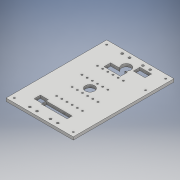
# Autodesk Inventor part: 一枚目
Saved by Autodesk Inventor 2018 (Build 220112000, 112)
## iProperties
Created: 2018-08-15
Part Number: 一枚目
Material: 一般
Document SubType Name: Modeling
Designer: shun2
Density: 1 g/cm^3
Appearance: 既定
Author: shun2
Autodesk Inventor part; units mm, degrees
(part 1 of 2)
ref_plane "YZ Plane" through (0, 0, 0) normal (1, 0, 0) x (0, 1, 0)
ref_plane "XZ Plane" through (0, 0, 0) normal (0, 1, 0) x (-1, 0, 0)
ref_plane "XY Plane" through (0, 0, 0) normal (0, 0, 1) x (1, 0, 0)
sketch "スケッチ2" plane through (0, 0, 0) normal (0, 0, 1) x (1, 0, 0)
  line L0 (0.0414, 0.0414) -> (130.0414, 0.0414)
  line L1 (130.0414, 0.0414) -> (130.0414, 194.7653)
  line L2 (130.0414, 194.7653) -> (0.0414, 194.7653)
  line L3 (0.0414, 194.7653) -> (0.0414, 0.0414)
  circle A0 centre (78.0414, 186.7653) radius 2.15
  circle A1 centre (92.0414, 186.7653) radius 2.15
  circle A2 centre (52.0414, 186.7653) radius 2.15
  circle A3 centre (38.0414, 186.7653) radius 2.15
  circle A4 centre (78.0414, 8.0414) radius 2.15
  circle A5 centre (92.0414, 8.0414) radius 2.15
  circle A6 centre (52.0414, 8.0414) radius 2.15
  circle A7 centre (38.0414, 8.0414) radius 2.15
  circle A8 centre (95.5414, 52.4033) radius 1.6
  circle A9 centre (45.5414, 52.4033) radius 1.6
  circle A10 centre (55.5414, 52.4033) radius 1.6
  circle A11 centre (65.5414, 52.4033) radius 1.6
  circle A12 centre (75.5414, 52.4033) radius 1.6
  circle A13 centre (85.5414, 52.4033) radius 1.6
  circle A14 centre (95.5414, 82.4033) radius 1.6
  circle A15 centre (45.5414, 82.4033) radius 1.6
  circle A16 centre (55.5414, 82.4033) radius 1.6
  circle A17 centre (65.5414, 82.4033) radius 1.6
  circle A18 centre (75.5414, 82.4033) radius 1.6
  circle A19 centre (85.5414, 82.4033) radius 1.6
  circle A20 centre (34.5414, 142.4033) radius 1.6
  circle A21 centre (84.5414, 142.4033) radius 1.6
  circle A22 centre (74.5414, 142.4033) radius 1.6
  circle A23 centre (64.5414, 142.4033) radius 1.6
  circle A24 centre (54.5414, 142.4033) radius 1.6
  circle A25 centre (44.5414, 142.4033) radius 1.6
  circle A26 centre (34.5414, 112.4033) radius 1.6
  circle A27 centre (84.5414, 112.4033) radius 1.6
  circle A28 centre (74.5414, 112.4033) radius 1.6
  circle A29 centre (64.5414, 112.4033) radius 1.6
  circle A30 centre (54.5414, 112.4033) radius 1.6
  circle A31 centre (44.5414, 112.4033) radius 1.6
  circle A32 centre (8.0414, 186.7653) radius 1.6
  circle A33 centre (122.0414, 186.7653) radius 1.6
  circle A34 centre (122.0414, 8.0414) radius 1.6
  circle A35 centre (8.0414, 8.0414) radius 1.6
  circle A36 centre (122.0414, 147.7653) radius 1.6
  line L4 (130.0414, 194.7653) -> (0.0414, 194.7653)
  line L5 (0.0414, 194.7653) -> (0.0414, 0.0414)
  line L6 (0.0414, 0.0414) -> (130.0414, 0.0414)
  line L7 (130.0414, 0.0414) -> (130.0414, 194.7653)
  circle A37 centre (92.0414, 186.7653) radius 2.15
  circle A38 centre (78.0414, 186.7653) radius 2.15
  circle A39 centre (52.0414, 186.7653) radius 2.15
  circle A40 centre (38.0414, 186.7653) radius 2.15
  circle A41 centre (92.0414, 8.0414) radius 2.15
  circle A42 centre (78.0414, 8.0414) radius 2.15
  circle A43 centre (52.0414, 8.0414) radius 2.15
  circle A44 centre (38.0414, 8.0414) radius 2.15
  circle A45 centre (84.5414, 142.4033) radius 1.6
  circle A46 centre (74.5414, 142.4033) radius 1.6
  circle A47 centre (64.5414, 142.4033) radius 1.6
  circle A48 centre (54.5414, 142.4033) radius 1.6
  circle A49 centre (44.5414, 142.4033) radius 1.6
  circle A50 centre (34.5414, 142.4033) radius 1.6
  circle A51 centre (84.5414, 112.4033) radius 1.6
  circle A52 centre (74.5414, 112.4033) radius 1.6
  circle A53 centre (64.5414, 112.4033) radius 1.6
  circle A54 centre (54.5414, 112.4033) radius 1.6
  circle A55 centre (44.5414, 112.4033) radius 1.6
  circle A56 centre (34.5414, 112.4033) radius 1.6
  circle A57 centre (95.5414, 82.4033) radius 1.6
  circle A58 centre (85.5414, 82.4033) radius 1.6
  circle A59 centre (75.5414, 82.4033) radius 1.6
  circle A60 centre (65.5414, 82.4033) radius 1.6
  circle A61 centre (55.5414, 82.4033) radius 1.6
  circle A62 centre (45.5414, 82.4033) radius 1.6
  circle A63 centre (95.5414, 52.4033) radius 1.6
  circle A64 centre (85.5414, 52.4033) radius 1.6
  circle A65 centre (75.5414, 52.4033) radius 1.6
  circle A66 centre (65.5414, 52.4033) radius 1.6
  circle A67 centre (55.5414, 52.4033) radius 1.6
  circle A68 centre (45.5414, 82.4033) radius 1.6
  circle A69 centre (45.5414, 52.4033) radius 1.6
  circle A70 centre (8.0414, 186.7653) radius 1.6
  circle A71 centre (122.0414, 186.7653) radius 1.6
  circle A72 centre (122.0414, 147.7653) radius 1.6
  circle A73 centre (122.0414, 8.0414) radius 1.6
  circle A74 centre (8.0414, 8.0414) radius 1.6
  arc A75 (69.6765, 160.0343) -> (65, 176.7239) centre (65, 167.7239) ccw
  arc A76 (65, 176.7239) -> (60.3235, 160.0343) centre (65, 167.7239) ccw
  line L8 (83.4433, 173.4847) -> (95.4433, 173.4847)
  arc A77 (95.4433, 173.453) -> (95.4433, 173.5164) centre (95.4433, 173.4847) ccw
  arc A78 (83.4433, 173.5164) -> (83.4433, 173.453) centre (83.4433, 173.4847) ccw
  line L9 (95.4433, 173.4847) -> (95.4433, 176.9847)
  arc A79 (95.4751, 176.9847) -> (95.4116, 176.9847) centre (95.4434, 176.9847) ccw
  arc A80 (95.4116, 173.4847) -> (95.4751, 173.4847) centre (95.4434, 173.4847) ccw
  line L10 (95.4433, 176.9847) -> (83.4433, 176.9847)
  arc A81 (83.4433, 177.0164) -> (83.4433, 176.953) centre (83.4433, 176.9847) ccw
  arc A82 (95.4433, 176.953) -> (95.4433, 177.0164) centre (95.4433, 176.9847) ccw
  line L11 (83.4433, 176.9847) -> (83.4433, 173.4847)
  arc A83 (83.4116, 173.4847) -> (83.4751, 173.4847) centre (83.4434, 173.4847) ccw
  arc A84 (83.4751, 176.9847) -> (83.4116, 176.9847) centre (83.4434, 176.9847) ccw
  line L12 (56.515, 150.7744) -> (56.515, 152.1714)
  arc A85 (56.5531, 152.1714) -> (56.4769, 152.1714) centre (56.515, 152.1714) ccw
  arc A86 (56.4769, 150.7744) -> (56.5531, 150.7744) centre (56.515, 150.7744) ccw
  line L13 (46.355, 158.2674) -> (56.515, 158.2674)
  arc A87 (56.515, 158.2293) -> (56.515, 158.3055) centre (56.515, 158.2674) ccw
  arc A88 (46.355, 158.3055) -> (46.355, 158.2293) centre (46.355, 158.2674) ccw
  line L14 (46.355, 158.2674) -> (46.355, 156.4894)
  arc A89 (46.3169, 156.4894) -> (46.3931, 156.4894) centre (46.355, 156.4894) ccw
  arc A90 (46.3931, 158.2674) -> (46.3169, 158.2674) centre (46.355, 158.2674) ccw
  line L15 (56.515, 150.7744) -> (46.355, 150.7744)
  arc A91 (46.355, 150.8125) -> (46.355, 150.7363) centre (46.355, 150.7744) ccw
  arc A92 (56.515, 150.7363) -> (56.515, 150.8125) centre (56.515, 150.7744) ccw
  line L16 (56.515, 157.3784) -> (57.023, 157.5054)
  arc A93 (57.0322, 157.4684) -> (57.0138, 157.5424) centre (57.023, 157.5054) ccw
  arc A94 (56.5058, 157.4154) -> (56.5242, 157.3414) centre (56.515, 157.3784) ccw
  line L17 (56.515, 157.3784) -> (56.515, 158.2674)
  arc A95 (56.5531, 158.2674) -> (56.4769, 158.2674) centre (56.515, 158.2674) ccw
  arc A96 (56.4769, 157.3784) -> (56.5531, 157.3784) centre (56.515, 157.3784) ccw
  line L18 (57.023, 157.5054) -> (57.023, 156.3624)
  arc A97 (56.9849, 156.3624) -> (57.0611, 156.3624) centre (57.023, 156.3624) ccw
  arc A98 (57.0611, 157.5054) -> (56.9849, 157.5054) centre (57.023, 157.5054) ccw
  line L19 (57.023, 156.3624) -> (56.515, 156.4894)
  arc A99 (56.5242, 156.5264) -> (56.5058, 156.4524) centre (56.515, 156.4894) ccw
  arc A100 (57.0138, 156.3254) -> (57.0322, 156.3994) centre (57.023, 156.3624) ccw
  line L20 (56.515, 156.4894) -> (56.515, 157.3784)
  arc A101 (56.5531, 157.3784) -> (56.4769, 157.3784) centre (56.515, 157.3784) ccw
  arc A102 (56.4769, 156.4894) -> (56.5531, 156.4894) centre (56.515, 156.4894) ccw
  line L21 (56.515, 156.4894) -> (46.355, 156.4894)
  arc A103 (46.355, 156.5275) -> (46.355, 156.4513) centre (46.355, 156.4894) ccw
  arc A104 (56.515, 156.4513) -> (56.515, 156.5275) centre (56.515, 156.4894) ccw
  line L22 (46.355, 156.4894) -> (46.355, 152.1714)
  arc A105 (46.3169, 152.1714) -> (46.3931, 152.1714) centre (46.355, 152.1714) ccw
  arc A106 (46.3931, 156.4894) -> (46.3169, 156.4894) centre (46.355, 156.4894) ccw
  line L23 (56.515, 152.1714) -> (46.355, 152.1714)
  arc A107 (46.355, 152.2095) -> (46.355, 152.1333) centre (46.355, 152.1714) ccw
  arc A108 (56.515, 152.1333) -> (56.515, 152.2095) centre (56.515, 152.1714) ccw
  line L24 (56.515, 152.1714) -> (56.515, 156.4894)
  arc A109 (56.5531, 156.4894) -> (56.4769, 156.4894) centre (56.515, 156.4894) ccw
  arc A110 (56.4769, 152.1714) -> (56.5531, 152.1714) centre (56.515, 152.1714) ccw
  line L25 (46.355, 152.1714) -> (46.355, 150.7744)
  arc A111 (46.3169, 150.7744) -> (46.3931, 150.7744) centre (46.355, 150.7744) ccw
  arc A112 (46.3931, 152.1714) -> (46.3169, 152.1714) centre (46.355, 152.1714) ccw
  line L26 (60.565, 151.81) -> (60.565, 156.89)
  arc A113 (60.5968, 156.89) -> (60.5333, 156.89) centre (60.5651, 156.89) ccw
  arc A114 (60.5333, 151.81) -> (60.5968, 151.81) centre (60.5651, 151.81) ccw
  line L27 (60.565, 156.89) -> (61.835, 156.89)
  arc A115 (61.835, 156.8583) -> (61.835, 156.9218) centre (61.835, 156.8901) ccw
  arc A116 (60.565, 156.9218) -> (60.565, 156.8583) centre (60.565, 156.8901) ccw
  line L28 (61.835, 156.89) -> (69.455, 156.89)
  arc A117 (69.455, 156.8583) -> (69.455, 156.9218) centre (69.455, 156.8901) ccw
  arc A118 (61.835, 156.9218) -> (61.835, 156.8583) centre (61.835, 156.8901) ccw
  line L29 (69.455, 156.89) -> (70.725, 156.89)
  arc A119 (70.725, 156.8583) -> (70.725, 156.9218) centre (70.725, 156.8901) ccw
  arc A120 (69.455, 156.9218) -> (69.455, 156.8583) centre (69.455, 156.8901) ccw
  line L30 (70.725, 156.89) -> (70.725, 151.81)
  arc A121 (70.6933, 151.81) -> (70.7568, 151.81) centre (70.725, 151.81) ccw
  arc A122 (70.7568, 156.89) -> (70.6933, 156.89) centre (70.725, 156.89) ccw
  line L31 (70.725, 151.81) -> (60.565, 151.81)
  arc A123 (60.565, 151.8417) -> (60.565, 151.7783) centre (60.565, 151.81) ccw
  arc A124 (70.725, 151.7783) -> (70.725, 151.8417) centre (70.725, 151.81) ccw
  line L32 (61.835, 156.89) -> (61.835, 155.62)
  arc A125 (61.8032, 155.62) -> (61.8668, 155.62) centre (61.835, 155.62) ccw
  arc A126 (61.8668, 156.89) -> (61.8032, 156.89) centre (61.835, 156.89) ccw
  line L33 (61.835, 155.62) -> (69.455, 155.62)
  arc A127 (69.455, 155.5883) -> (69.455, 155.6517) centre (69.455, 155.62) ccw
  arc A128 (61.835, 155.6517) -> (61.835, 155.5883) centre (61.835, 155.62) ccw
  line L34 (69.455, 155.62) -> (69.455, 156.89)
  arc A129 (69.4868, 156.89) -> (69.4232, 156.89) centre (69.455, 156.89) ccw
  arc A130 (69.4232, 155.62) -> (69.4868, 155.62) centre (69.455, 155.62) ccw
  arc A131 (93.9433, 174.5922) -> (93.9433, 175.1172) centre (93.9433, 174.8547) ccw
  arc A132 (93.9433, 175.1172) -> (93.9433, 174.5922) centre (93.9433, 174.8547) ccw
  arc A133 (93.9433, 174.5922) -> (93.9433, 175.1172) centre (93.9433, 174.8547) ccw
  arc A134 (93.9433, 175.1172) -> (93.9433, 174.5922) centre (93.9433, 174.8547) ccw
  arc A135 (92.4433, 174.5922) -> (92.4433, 175.1172) centre (92.4433, 174.8547) ccw
  arc A136 (92.4433, 175.1172) -> (92.4433, 174.5922) centre (92.4433, 174.8547) ccw
  arc A137 (92.4433, 174.5922) -> (92.4433, 175.1172) centre (92.4433, 174.8547) ccw
  arc A138 (92.4433, 175.1172) -> (92.4433, 174.5922) centre (92.4433, 174.8547) ccw
  arc A139 (90.9433, 174.5922) -> (90.9433, 175.1172) centre (90.9433, 174.8547) ccw
  arc A140 (90.9433, 175.1172) -> (90.9433, 174.5922) centre (90.9433, 174.8547) ccw
  arc A141 (90.9433, 174.5922) -> (90.9433, 175.1172) centre (90.9433, 174.8547) ccw
  arc A142 (90.9433, 175.1172) -> (90.9433, 174.5922) centre (90.9433, 174.8547) ccw
  arc A143 (89.4433, 174.5922) -> (89.4433, 175.1172) centre (89.4433, 174.8547) ccw
  arc A144 (89.4433, 175.1172) -> (89.4433, 174.5922) centre (89.4433, 174.8547) ccw
  arc A145 (89.4433, 174.5922) -> (89.4433, 175.1172) centre (89.4433, 174.8547) ccw
  arc A146 (89.4433, 175.1172) -> (89.4433, 174.5922) centre (89.4433, 174.8547) ccw
  arc A147 (87.9433, 174.5922) -> (87.9433, 175.1172) centre (87.9433, 174.8547) ccw
  arc A148 (87.9433, 175.1172) -> (87.9433, 174.5922) centre (87.9433, 174.8547) ccw
  arc A149 (87.9433, 174.5922) -> (87.9433, 175.1172) centre (87.9433, 174.8547) ccw
  arc A150 (87.9433, 175.1172) -> (87.9433, 174.5922) centre (87.9433, 174.8547) ccw
  arc A151 (86.4433, 174.5922) -> (86.4433, 175.1172) centre (86.4433, 174.8547) ccw
  arc A152 (86.4433, 175.1172) -> (86.4433, 174.5922) centre (86.4433, 174.8547) ccw
  arc A153 (86.4433, 174.5922) -> (86.4433, 175.1172) centre (86.4433, 174.8547) ccw
  arc A154 (86.4433, 175.1172) -> (86.4433, 174.5922) centre (86.4433, 174.8547) ccw
  arc A155 (84.9433, 174.5922) -> (84.9433, 175.1172) centre (84.9433, 174.8547) ccw
  arc A156 (84.9433, 175.1172) -> (84.9433, 174.5922) centre (84.9433, 174.8547) ccw
  arc A157 (84.9433, 174.5922) -> (84.9433, 175.1172) centre (84.9433, 174.8547) ccw
  arc A158 (84.9433, 175.1172) -> (84.9433, 174.5922) centre (84.9433, 174.8547) ccw
  line L35 (51.935, 154.8304) -> (50.935, 154.8304)
  line L36 (50.935, 154.8304) -> (50.935, 153.8304)
  line L37 (50.935, 153.8304) -> (51.935, 153.8304)
  line L38 (51.935, 153.8304) -> (51.935, 154.8304)
  line L39 (53.9496, 153.3398) -> (53.9496, 155.321)
  arc A159 (54.4449, 155.321) -> (53.4543, 155.321) centre (53.9496, 155.321) ccw
  arc A160 (53.4543, 153.3398) -> (54.4449, 153.3398) centre (53.9496, 153.3398) ccw
  line L40 (53.9496, 153.3398) -> (53.9496, 155.321)
  arc A161 (54.4449, 155.321) -> (53.4543, 155.321) centre (53.9496, 155.321) ccw
  arc A162 (53.4543, 153.3398) -> (54.4449, 153.3398) centre (53.9496, 153.3398) ccw
  line L41 (48.9204, 153.3398) -> (48.9204, 155.321)
  arc A163 (49.4157, 155.321) -> (48.4251, 155.321) centre (48.9204, 155.321) ccw
  arc A164 (48.4251, 153.3398) -> (49.4157, 153.3398) centre (48.9204, 153.3398) ccw
  line L42 (48.9204, 153.3398) -> (48.9204, 155.321)
  arc A165 (49.4157, 155.321) -> (48.4251, 155.321) centre (48.9204, 155.321) ccw
  arc A166 (48.4251, 153.3398) -> (49.4157, 153.3398) centre (48.9204, 153.3398) ccw
  arc A167 (63.105, 153.9) -> (63.105, 154.8) centre (63.105, 154.35) ccw
  arc A168 (63.105, 154.8) -> (63.105, 153.9) centre (63.105, 154.35) ccw
  arc A169 (63.105, 153.9) -> (63.105, 154.8) centre (63.105, 154.35) ccw
  arc A170 (63.105, 154.8) -> (63.105, 153.9) centre (63.105, 154.35) ccw
  arc A171 (65.645, 153.9) -> (65.645, 154.8) centre (65.645, 154.35) ccw
  arc A172 (65.645, 154.8) -> (65.645, 153.9) centre (65.645, 154.35) ccw
  arc A173 (65.645, 153.9) -> (65.645, 154.8) centre (65.645, 154.35) ccw
  arc A174 (65.645, 154.8) -> (65.645, 153.9) centre (65.645, 154.35) ccw
  arc A175 (68.185, 153.9) -> (68.185, 154.8) centre (68.185, 154.35) ccw
  arc A176 (68.185, 154.8) -> (68.185, 153.9) centre (68.185, 154.35) ccw
  arc A177 (68.185, 153.9) -> (68.185, 154.8) centre (68.185, 154.35) ccw
  arc A178 (68.185, 154.8) -> (68.185, 153.9) centre (68.185, 154.35) ccw
  line L43 (74.3631, 160.0343) -> (74.3631, 147.2613)
  line L44 (74.3631, 147.2613) -> (42.3354, 147.2613)
  line L45 (42.3354, 147.2613) -> (42.3354, 160.0343)
  line L46 (78, 180.9909) -> (100.5174, 180.9909)
  line L47 (100.5174, 180.9909) -> (100.5174, 168.379)
  line L48 (100.5174, 168.379) -> (78, 168.379)
  line L49 (78, 168.379) -> (78, 180.9909)
  arc A179 (69.6765, 160.0343) -> (60.3235, 160.0343) centre (65, 167.7239) ccw
  line L50 (42.3354, 160.0343) -> (60.3235, 160.0343)
  line L51 (69.6765, 160.0343) -> (74.3631, 160.0343)
  arc A180 (65, 88.362) -> (65, 106.362) centre (65, 97.362) ccw
  arc A181 (65, 106.362) -> (65, 88.362) centre (65, 97.362) ccw
  circle A182 centre (65, 97.362) radius 9
  line L52 (89.7664, 26.5952) -> (89.6098, 26.5952)
  arc A183 (89.6098, 26.6143) -> (89.6098, 26.5762) centre (89.6098, 26.5953) ccw
  arc A184 (89.7664, 26.5762) -> (89.7664, 26.6143) centre (89.7664, 26.5953) ccw
  line L53 (89.6098, 26.5952) -> (89.6098, 26.0731)
  arc A185 (89.5907, 26.0731) -> (89.6288, 26.0731) centre (89.6097, 26.0731) ccw
  arc A186 (89.6288, 26.5952) -> (89.5907, 26.5952) centre (89.6097, 26.5952) ccw
  line L54 (89.6098, 26.0731) -> (89.9231, 26.0731)
  arc A187 (89.9231, 26.0541) -> (89.9231, 26.0922) centre (89.9231, 26.0731) ccw
  arc A188 (89.6098, 26.0922) -> (89.6098, 26.0541) centre (89.6098, 26.0731) ccw
  arc A189 (89.9231, 26.0731) -> (90.1319, 26.2819) centre (89.9231, 26.2819) ccw
  arc A190 (89.9231, 26.0922) -> (89.9231, 26.0541) centre (89.9231, 26.0731) ccw
  arc A191 (90.1509, 26.2819) -> (90.1129, 26.2819) centre (90.1319, 26.2819) ccw
  line L55 (90.1319, 26.2819) -> (90.1319, 26.8041)
  arc A192 (90.1509, 26.8041) -> (90.1129, 26.8041) centre (90.1319, 26.8041) ccw
  arc A193 (90.1129, 26.2819) -> (90.1509, 26.2819) centre (90.1319, 26.2819) ccw
  arc A194 (90.1319, 26.8041) -> (89.9231, 27.0129) centre (89.9231, 26.8041) ccw
  arc A195 (90.1129, 26.8041) -> (90.1509, 26.8041) centre (90.1319, 26.8041) ccw
  arc A196 (89.9231, 27.0319) -> (89.9231, 26.9938) centre (89.9231, 27.0129) ccw
  line L56 (89.9231, 27.0129) -> (89.6098, 27.0129)
  arc A197 (89.6098, 27.032) -> (89.6098, 26.9939) centre (89.6098, 27.013) ccw
  arc A198 (89.9231, 26.9939) -> (89.9231, 27.032) centre (89.9231, 27.013) ccw
  arc A199 (84.5298, 26.2819) -> (84.7386, 26.0731) centre (84.7386, 26.2819) ccw
  arc A200 (84.5488, 26.2819) -> (84.5107, 26.2819) centre (84.5298, 26.2819) ccw
  arc A201 (84.7386, 26.0541) -> (84.7386, 26.0922) centre (84.7386, 26.0731) ccw
  arc A202 (84.7386, 26.0731) -> (85.0519, 26.2036) centre (84.7387, 26.5143) ccw
  arc A203 (84.7386, 26.0921) -> (84.7386, 26.0541) centre (84.7386, 26.0731) ccw
  arc A204 (85.0654, 26.1902) -> (85.0384, 26.217) centre (85.0519, 26.2036) ccw
  arc A205 (85.0258, 26.8041) -> (84.817, 27.0129) centre (84.817, 26.8041) ccw
  arc A206 (85.0067, 26.8041) -> (85.0448, 26.8041) centre (85.0257, 26.8041) ccw
  arc A207 (84.817, 27.032) -> (84.817, 26.9939) centre (84.817, 27.013) ccw
  arc A208 (84.817, 27.0129) -> (84.582, 26.9346) centre (84.8169, 26.6213) ccw
  arc A209 (84.817, 26.9939) -> (84.8169, 27.032) centre (84.817, 27.013) ccw
  arc A210 (84.5706, 26.9498) -> (84.5934, 26.9193) centre (84.582, 26.9346) ccw
  arc A211 (84.9214, 26.6213) -> (85.0258, 26.8041) centre (84.8137, 26.804) ccw
  arc A212 (84.9117, 26.6377) -> (84.931, 26.6049) centre (84.9213, 26.6213) ccw
  arc A213 (85.0448, 26.8041) -> (85.0067, 26.8041) centre (85.0257, 26.8041) ccw
  arc A214 (84.6342, 26.4647) -> (84.5298, 26.2819) centre (84.7419, 26.282) ccw
  arc A215 (84.6439, 26.4483) -> (84.6245, 26.4811) centre (84.6342, 26.4647) ccw
  arc A216 (84.5107, 26.2819) -> (84.5488, 26.2819) centre (84.5298, 26.2819) ccw
  line L57 (84.6342, 26.4647) -> (84.9214, 26.6213)
  arc A217 (84.9305, 26.6046) -> (84.9123, 26.638) centre (84.9214, 26.6213) ccw
  arc A218 (84.6251, 26.4814) -> (84.6433, 26.448) centre (84.6342, 26.4647) ccw
  line L58 (84.0898, 27.0129) -> (84.0898, 26.0731)
  arc A219 (84.0708, 26.0731) -> (84.1089, 26.0731) centre (84.0899, 26.0731) ccw
  arc A220 (84.1089, 27.0129) -> (84.0708, 27.0129) centre (84.0899, 27.0129) ccw
  line L59 (84.1942, 26.0731) -> (83.9854, 26.0731)
  arc A221 (83.9854, 26.0922) -> (83.9854, 26.0541) centre (83.9854, 26.0731) ccw
  arc A222 (84.1942, 26.0541) -> (84.1942, 26.0922) centre (84.1942, 26.0731) ccw
  line L60 (84.1942, 27.0129) -> (83.9854, 27.0129)
  arc A223 (83.9854, 27.032) -> (83.9854, 26.9939) centre (83.9854, 27.013) ccw
  arc A224 (84.1942, 26.9939) -> (84.1942, 27.032) centre (84.1942, 27.013) ccw
  line L61 (83.2234, 26.5952) -> (83.0668, 26.5952)
  arc A225 (83.0668, 26.6143) -> (83.0668, 26.5762) centre (83.0668, 26.5953) ccw
  arc A226 (83.2234, 26.5762) -> (83.2234, 26.6143) centre (83.2234, 26.5953) ccw
  line L62 (83.0668, 26.5952) -> (83.0668, 26.0731)
  arc A227 (83.0477, 26.0731) -> (83.0858, 26.0731) centre (83.0668, 26.0731) ccw
  arc A228 (83.0858, 26.5952) -> (83.0477, 26.5952) centre (83.0668, 26.5952) ccw
  line L63 (83.0668, 26.0731) -> (83.38, 26.0731)
  arc A229 (83.38, 26.0541) -> (83.38, 26.0922) centre (83.38, 26.0731) ccw
  arc A230 (83.0668, 26.0922) -> (83.0668, 26.0541) centre (83.0668, 26.0731) ccw
  arc A231 (83.38, 26.0731) -> (83.5889, 26.2819) centre (83.38, 26.282) ccw
  arc A232 (83.38, 26.0922) -> (83.38, 26.0541) centre (83.38, 26.0731) ccw
  arc A233 (83.6079, 26.2819) -> (83.5698, 26.2819) centre (83.5889, 26.2819) ccw
  line L64 (83.5889, 26.2819) -> (83.5889, 26.8041)
  arc A234 (83.6079, 26.8041) -> (83.5698, 26.8041) centre (83.5889, 26.8041) ccw
  arc A235 (83.5698, 26.2819) -> (83.6079, 26.2819) centre (83.5889, 26.2819) ccw
  arc A236 (83.5889, 26.8041) -> (83.38, 27.0129) centre (83.38, 26.804) ccw
  arc A237 (83.5698, 26.8041) -> (83.6079, 26.8041) centre (83.5889, 26.8041) ccw
  arc A238 (83.38, 27.0319) -> (83.38, 26.9938) centre (83.38, 27.0129) ccw
  line L65 (83.38, 27.0129) -> (83.0668, 27.0129)
  arc A239 (83.0668, 27.032) -> (83.0668, 26.9939) centre (83.0668, 27.013) ccw
  arc A240 (83.38, 26.9939) -> (83.38, 27.032) centre (83.38, 27.013) ccw
  line L66 (31.115, 35.941) -> (31.115, 34.544)
  arc A241 (31.0769, 34.544) -> (31.1531, 34.544) centre (31.115, 34.544) ccw
  arc A242 (31.1531, 35.941) -> (31.0769, 35.941) centre (31.115, 35.941) ccw
  line L67 (41.275, 28.448) -> (31.115, 28.448)
  arc A243 (31.115, 28.4861) -> (31.115, 28.4099) centre (31.115, 28.448) ccw
  arc A244 (41.275, 28.4099) -> (41.275, 28.4861) centre (41.275, 28.448) ccw
  line L68 (41.275, 28.448) -> (41.275, 30.226)
  arc A245 (41.3131, 30.226) -> (41.2369, 30.226) centre (41.275, 30.226) ccw
  arc A246 (41.2369, 28.448) -> (41.3131, 28.448) centre (41.275, 28.448) ccw
  line L69 (31.115, 35.941) -> (41.275, 35.941)
  arc A247 (41.275, 35.9029) -> (41.275, 35.9791) centre (41.275, 35.941) ccw
  arc A248 (31.115, 35.9791) -> (31.115, 35.9029) centre (31.115, 35.941) ccw
  line L70 (31.115, 29.337) -> (30.607, 29.21)
  arc A249 (30.5978, 29.247) -> (30.6162, 29.173) centre (30.607, 29.21) ccw
  arc A250 (31.1242, 29.3) -> (31.1058, 29.374) centre (31.115, 29.337) ccw
  line L71 (31.115, 29.337) -> (31.115, 28.448)
  arc A251 (31.0769, 28.448) -> (31.1531, 28.448) centre (31.115, 28.448) ccw
  arc A252 (31.1531, 29.337) -> (31.0769, 29.337) centre (31.115, 29.337) ccw
  line L72 (30.607, 29.21) -> (30.607, 30.353)
  arc A253 (30.6451, 30.353) -> (30.5689, 30.353) centre (30.607, 30.353) ccw
  arc A254 (30.5689, 29.21) -> (30.6451, 29.21) centre (30.607, 29.21) ccw
  line L73 (30.607, 30.353) -> (31.115, 30.226)
  arc A255 (31.1058, 30.189) -> (31.1242, 30.263) centre (31.115, 30.226) ccw
  arc A256 (30.6162, 30.39) -> (30.5978, 30.316) centre (30.607, 30.353) ccw
  line L74 (31.115, 30.226) -> (31.115, 29.337)
  arc A257 (31.0769, 29.337) -> (31.1531, 29.337) centre (31.115, 29.337) ccw
  arc A258 (31.1531, 30.226) -> (31.0769, 30.226) centre (31.115, 30.226) ccw
  line L75 (31.115, 30.226) -> (41.275, 30.226)
  arc A259 (41.275, 30.1879) -> (41.275, 30.2641) centre (41.275, 30.226) ccw
  arc A260 (31.115, 30.2641) -> (31.115, 30.1879) centre (31.115, 30.226) ccw
  line L76 (41.275, 30.226) -> (41.275, 34.544)
  arc A261 (41.3131, 34.544) -> (41.2369, 34.544) centre (41.275, 34.544) ccw
  arc A262 (41.2369, 30.226) -> (41.3131, 30.226) centre (41.275, 30.226) ccw
  line L77 (31.115, 34.544) -> (41.275, 34.544)
  arc A263 (41.275, 34.5059) -> (41.275, 34.5821) centre (41.275, 34.544) ccw
  arc A264 (31.115, 34.5821) -> (31.115, 34.5059) centre (31.115, 34.544) ccw
  line L78 (31.115, 34.544) -> (31.115, 30.226)
  arc A265 (31.0769, 30.226) -> (31.1531, 30.226) centre (31.115, 30.226) ccw
  arc A266 (31.1531, 34.544) -> (31.0769, 34.544) centre (31.115, 34.544) ccw
  line L79 (41.275, 34.544) -> (41.275, 35.941)
  arc A267 (41.3131, 35.941) -> (41.2369, 35.941) centre (41.275, 35.941) ccw
  arc A268 (41.2369, 34.544) -> (41.3131, 34.544) centre (41.275, 34.544) ccw
  line L80 (32.2933, 29.5896) -> (32.0534, 29.7815)
  arc A269 (32.0732, 29.8063) -> (32.0336, 29.7567) centre (32.0534, 29.7815) ccw
  arc A270 (32.2734, 29.5648) -> (32.3131, 29.6144) centre (32.2933, 29.5896) ccw
  line L81 (32.0534, 29.7815) -> (32.0534, 28.9179)
  arc A271 (32.0216, 28.9179) -> (32.0851, 28.9179) centre (32.0533, 28.9179) ccw
  arc A272 (32.0851, 29.7815) -> (32.0216, 29.7815) centre (32.0533, 29.7815) ccw
  line L82 (32.2933, 28.9179) -> (31.8135, 28.9179)
  arc A273 (31.8135, 28.9497) -> (31.8135, 28.8862) centre (31.8135, 28.918) ccw
  arc A274 (32.2933, 28.8862) -> (32.2933, 28.9497) centre (32.2933, 28.918) ccw
  arc A275 (37.1094, 29.7815) -> (36.8935, 29.5656) centre (37.1094, 29.5656) ccw
  arc A276 (37.1094, 29.7498) -> (37.1094, 29.8133) centre (37.1094, 29.7816) ccw
  arc A277 (36.8618, 29.5656) -> (36.9253, 29.5656) centre (36.8936, 29.5656) ccw
  arc A278 (37.3733, 29.5896) -> (37.1094, 29.7815) centre (37.1094, 29.5041) ccw
  arc A279 (37.3431, 29.5798) -> (37.4035, 29.5994) centre (37.3733, 29.5896) ccw
  arc A280 (37.1094, 29.8132) -> (37.1094, 29.7498) centre (37.1094, 29.7815) ccw
  arc A281 (36.8935, 29.5656) -> (36.9655, 29.3977) centre (37.1253, 29.5656) ccw
  arc A282 (36.9252, 29.5656) -> (36.8618, 29.5656) centre (36.8935, 29.5656) ccw
  arc A283 (36.9436, 29.3747) -> (36.9874, 29.4207) centre (36.9655, 29.3977) ccw
  line L83 (36.9655, 29.3977) -> (37.3733, 28.9179)
  arc A284 (37.3491, 28.8973) -> (37.3975, 28.9385) centre (37.3733, 28.9179) ccw
  arc A285 (36.9897, 29.4182) -> (36.9413, 29.3771) centre (36.9655, 29.3976) ccw
  line L84 (37.3733, 28.9179) -> (36.8935, 28.9179)
  arc A286 (36.8935, 28.9497) -> (36.8935, 28.8862) centre (36.8935, 28.918) ccw
  arc A287 (37.3733, 28.8862) -> (37.3733, 28.9497) centre (37.3733, 28.918) ccw
  arc A288 (38.7096, 28.829) -> (38.7096, 29.845) centre (38.7096, 29.337) ccw
  arc A289 (38.7096, 29.845) -> (38.7096, 28.829) centre (38.7096, 29.337) ccw
  arc A290 (33.6804, 28.829) -> (33.6804, 29.845) centre (33.6804, 29.337) ccw
  arc A291 (33.6804, 29.845) -> (33.6804, 28.829) centre (33.6804, 29.337) ccw
  line L85 (47.085, 27.46) -> (48.355, 27.46)
  arc A292 (48.355, 27.4219) -> (48.355, 27.4981) centre (48.355, 27.46) ccw
  arc A293 (47.085, 27.4981) -> (47.085, 27.4219) centre (47.085, 27.46) ccw
  line L86 (48.355, 27.46) -> (48.99, 28.095)
  arc A294 (49.0169, 28.0681) -> (48.9631, 28.1219) centre (48.99, 28.095) ccw
  arc A295 (48.3281, 27.4869) -> (48.3819, 27.4331) centre (48.355, 27.46) ccw
  line L87 (48.99, 29.365) -> (48.355, 30)
  arc A296 (48.3819, 30.0269) -> (48.3281, 29.9731) centre (48.355, 30) ccw
  arc A297 (48.9631, 29.3381) -> (49.0169, 29.3919) centre (48.99, 29.365) ccw
  line L88 (48.99, 28.095) -> (49.625, 27.46)
  arc A298 (49.5981, 27.4331) -> (49.6519, 27.4869) centre (49.625, 27.46) ccw
  arc A299 (49.0169, 28.1219) -> (48.9631, 28.0681) centre (48.99, 28.095) ccw
  line L89 (49.625, 27.46) -> (50.895, 27.46)
  arc A300 (50.895, 27.4219) -> (50.895, 27.4981) centre (50.895, 27.46) ccw
  arc A301 (49.625, 27.4981) -> (49.625, 27.4219) centre (49.625, 27.46) ccw
  line L90 (50.895, 27.46) -> (51.53, 28.095)
  arc A302 (51.5569, 28.0681) -> (51.5031, 28.1219) centre (51.53, 28.095) ccw
  arc A303 (50.8681, 27.4869) -> (50.9219, 27.4331) centre (50.895, 27.46) ccw
  line L91 (51.53, 29.365) -> (50.895, 30)
  arc A304 (50.9219, 30.0269) -> (50.8681, 29.9731) centre (50.895, 30) ccw
  arc A305 (51.5031, 29.3381) -> (51.5569, 29.3919) centre (51.53, 29.365) ccw
  line L92 (50.895, 30) -> (49.625, 30)
  arc A306 (49.625, 30.0381) -> (49.625, 29.9619) centre (49.625, 30) ccw
  arc A307 (50.895, 29.9619) -> (50.895, 30.0381) centre (50.895, 30) ccw
  line L93 (49.625, 30) -> (48.99, 29.365)
  arc A308 (48.9631, 29.3919) -> (49.0169, 29.3381) centre (48.99, 29.365) ccw
  arc A309 (49.6519, 29.9731) -> (49.5981, 30.0269) centre (49.625, 30) ccw
  line L94 (46.45, 28.095) -> (46.45, 29.365)
  arc A310 (46.4881, 29.365) -> (46.4119, 29.365) centre (46.45, 29.365) ccw
  arc A311 (46.4119, 28.095) -> (46.4881, 28.095) centre (46.45, 28.095) ccw
  line L95 (47.085, 27.46) -> (46.45, 28.095)
  arc A312 (46.4769, 28.1219) -> (46.4231, 28.0681) centre (46.45, 28.095) ccw
  arc A313 (47.0581, 27.4331) -> (47.1119, 27.4869) centre (47.085, 27.46) ccw
  line L96 (46.45, 29.365) -> (47.085, 30)
  arc A314 (47.1119, 29.9731) -> (47.0581, 30.0269) centre (47.085, 30) ccw
  arc A315 (46.4231, 29.3919) -> (46.4769, 29.3381) centre (46.45, 29.365) ccw
  line L97 (48.355, 30) -> (47.085, 30)
  arc A316 (47.085, 30.0381) -> (47.085, 29.9619) centre (47.085, 30) ccw
  arc A317 (48.355, 29.9619) -> (48.355, 30.0381) centre (48.355, 30) ccw
  line L98 (51.53, 28.095) -> (52.165, 27.46)
  arc A318 (52.1381, 27.4331) -> (52.1919, 27.4869) centre (52.165, 27.46) ccw
  arc A319 (51.5569, 28.1219) -> (51.5031, 28.0681) centre (51.53, 28.095) ccw
  line L99 (52.165, 27.46) -> (53.435, 27.46)
  arc A320 (53.435, 27.4219) -> (53.435, 27.4981) centre (53.435, 27.46) ccw
  arc A321 (52.165, 27.4981) -> (52.165, 27.4219) centre (52.165, 27.46) ccw
  line L100 (53.435, 27.46) -> (54.07, 28.095)
  arc A322 (54.0969, 28.0681) -> (54.0431, 28.1219) centre (54.07, 28.095) ccw
  arc A323 (53.4081, 27.4869) -> (53.4619, 27.4331) centre (53.435, 27.46) ccw
  line L101 (54.07, 29.365) -> (53.435, 30)
  arc A324 (53.4619, 30.0269) -> (53.4081, 29.9731) centre (53.435, 30) ccw
  arc A325 (54.0431, 29.3381) -> (54.0969, 29.3919) centre (54.07, 29.365) ccw
  line L102 (53.435, 30) -> (52.165, 30)
  arc A326 (52.165, 30.0381) -> (52.165, 29.9619) centre (52.165, 30) ccw
  arc A327 (53.435, 29.9619) -> (53.435, 30.0381) centre (53.435, 30) ccw
  line L103 (52.165, 30) -> (51.53, 29.365)
  arc A328 (51.5031, 29.3919) -> (51.5569, 29.3381) centre (51.53, 29.365) ccw
  arc A329 (52.1919, 29.9731) -> (52.1381, 30.0269) centre (52.165, 30) ccw
  line L104 (54.705, 27.46) -> (55.975, 27.46)
  arc A330 (55.975, 27.4219) -> (55.975, 27.4981) centre (55.975, 27.46) ccw
  arc A331 (54.705, 27.4981) -> (54.705, 27.4219) centre (54.705, 27.46) ccw
  line L105 (55.975, 27.46) -> (56.61, 28.095)
  arc A332 (56.6369, 28.0681) -> (56.5831, 28.1219) centre (56.61, 28.095) ccw
  arc A333 (55.9481, 27.4869) -> (56.0019, 27.4331) centre (55.975, 27.46) ccw
  line L106 (56.61, 29.365) -> (55.975, 30)
  arc A334 (56.0019, 30.0269) -> (55.9481, 29.9731) centre (55.975, 30) ccw
  arc A335 (56.5831, 29.3381) -> (56.6369, 29.3919) centre (56.61, 29.365) ccw
  line L107 (56.61, 28.095) -> (57.245, 27.46)
  arc A336 (57.2181, 27.4331) -> (57.2719, 27.4869) centre (57.245, 27.46) ccw
  arc A337 (56.6369, 28.1219) -> (56.5831, 28.0681) centre (56.61, 28.095) ccw
  line L108 (57.245, 27.46) -> (58.515, 27.46)
  arc A338 (58.515, 27.4219) -> (58.515, 27.4981) centre (58.515, 27.46) ccw
  arc A339 (57.245, 27.4981) -> (57.245, 27.4219) centre (57.245, 27.46) ccw
  line L109 (58.515, 27.46) -> (59.15, 28.095)
  arc A340 (59.1769, 28.0681) -> (59.1231, 28.1219) centre (59.15, 28.095) ccw
  arc A341 (58.4881, 27.4869) -> (58.5419, 27.4331) centre (58.515, 27.46) ccw
  line L110 (59.15, 29.365) -> (58.515, 30)
  arc A342 (58.5419, 30.0269) -> (58.4881, 29.9731) centre (58.515, 30) ccw
  arc A343 (59.1231, 29.3381) -> (59.1769, 29.3919) centre (59.15, 29.365) ccw
  line L111 (58.515, 30) -> (57.245, 30)
  arc A344 (57.245, 30.0381) -> (57.245, 29.9619) centre (57.245, 30) ccw
  arc A345 (58.515, 29.9619) -> (58.515, 30.0381) centre (58.515, 30) ccw
  line L112 (57.245, 30) -> (56.61, 29.365)
  arc A346 (56.5831, 29.3919) -> (56.6369, 29.3381) centre (56.61, 29.365) ccw
  arc A347 (57.2719, 29.9731) -> (57.2181, 30.0269) centre (57.245, 30) ccw
  line L113 (54.705, 27.46) -> (54.07, 28.095)
  arc A348 (54.0969, 28.1219) -> (54.0431, 28.0681) centre (54.07, 28.095) ccw
  arc A349 (54.6781, 27.4331) -> (54.7319, 27.4869) centre (54.705, 27.46) ccw
  line L114 (54.07, 29.365) -> (54.705, 30)
  arc A350 (54.7319, 29.9731) -> (54.6781, 30.0269) centre (54.705, 30) ccw
  arc A351 (54.0431, 29.3919) -> (54.0969, 29.3381) centre (54.07, 29.365) ccw
  line L115 (55.975, 30) -> (54.705, 30)
  arc A352 (54.705, 30.0381) -> (54.705, 29.9619) centre (54.705, 30) ccw
  arc A353 (55.975, 29.9619) -> (55.975, 30.0381) centre (55.975, 30) ccw
  line L116 (59.15, 28.095) -> (59.785, 27.46)
  arc A354 (59.7581, 27.4331) -> (59.8119, 27.4869) centre (59.785, 27.46) ccw
  arc A355 (59.1769, 28.1219) -> (59.1231, 28.0681) centre (59.15, 28.095) ccw
  line L117 (59.785, 27.46) -> (61.055, 27.46)
  arc A356 (61.055, 27.4219) -> (61.055, 27.4981) centre (61.055, 27.46) ccw
  arc A357 (59.785, 27.4981) -> (59.785, 27.4219) centre (59.785, 27.46) ccw
  line L118 (61.055, 27.46) -> (61.69, 28.095)
  arc A358 (61.7169, 28.0681) -> (61.6631, 28.1219) centre (61.69, 28.095) ccw
  arc A359 (61.0281, 27.4869) -> (61.0819, 27.4331) centre (61.055, 27.46) ccw
  line L119 (61.69, 29.365) -> (61.055, 30)
  arc A360 (61.0819, 30.0269) -> (61.0281, 29.9731) centre (61.055, 30) ccw
  arc A361 (61.6631, 29.3381) -> (61.7169, 29.3919) centre (61.69, 29.365) ccw
  line L120 (61.055, 30) -> (59.785, 30)
  arc A362 (59.785, 30.0381) -> (59.785, 29.9619) centre (59.785, 30) ccw
  arc A363 (61.055, 29.9619) -> (61.055, 30.0381) centre (61.055, 30) ccw
  line L121 (59.785, 30) -> (59.15, 29.365)
  arc A364 (59.1231, 29.3919) -> (59.1769, 29.3381) centre (59.15, 29.365) ccw
  arc A365 (59.8119, 29.9731) -> (59.7581, 30.0269) centre (59.785, 30) ccw
  line L122 (62.325, 27.46) -> (63.595, 27.46)
  arc A366 (63.595, 27.4219) -> (63.595, 27.4981) centre (63.595, 27.46) ccw
  arc A367 (62.325, 27.4981) -> (62.325, 27.4219) centre (62.325, 27.46) ccw
  line L123 (63.595, 27.46) -> (64.23, 28.095)
  arc A368 (64.2569, 28.0681) -> (64.2031, 28.1219) centre (64.23, 28.095) ccw
  arc A369 (63.5681, 27.4869) -> (63.6219, 27.4331) centre (63.595, 27.46) ccw
  line L124 (64.23, 29.365) -> (63.595, 30)
  arc A370 (63.6219, 30.0269) -> (63.5681, 29.9731) centre (63.595, 30) ccw
  arc A371 (64.2031, 29.3381) -> (64.2569, 29.3919) centre (64.23, 29.365) ccw
  line L125 (64.23, 28.095) -> (64.865, 27.46)
  arc A372 (64.8381, 27.4331) -> (64.8919, 27.4869) centre (64.865, 27.46) ccw
  arc A373 (64.2569, 28.1219) -> (64.2031, 28.0681) centre (64.23, 28.095) ccw
  line L126 (64.865, 27.46) -> (66.135, 27.46)
  arc A374 (66.135, 27.4219) -> (66.135, 27.4981) centre (66.135, 27.46) ccw
  arc A375 (64.865, 27.4981) -> (64.865, 27.4219) centre (64.865, 27.46) ccw
  line L127 (66.135, 27.46) -> (66.77, 28.095)
  arc A376 (66.7969, 28.0681) -> (66.7431, 28.1219) centre (66.77, 28.095) ccw
  arc A377 (66.1081, 27.4869) -> (66.1619, 27.4331) centre (66.135, 27.46) ccw
  line L128 (66.77, 29.365) -> (66.135, 30)
  arc A378 (66.1619, 30.0269) -> (66.1081, 29.9731) centre (66.135, 30) ccw
  arc A379 (66.7431, 29.3381) -> (66.7969, 29.3919) centre (66.77, 29.365) ccw
  line L129 (66.135, 30) -> (64.865, 30)
  arc A380 (64.865, 30.0381) -> (64.865, 29.9619) centre (64.865, 30) ccw
  arc A381 (66.135, 29.9619) -> (66.135, 30.0381) centre (66.135, 30) ccw
  line L130 (64.865, 30) -> (64.23, 29.365)
  arc A382 (64.2031, 29.3919) -> (64.2569, 29.3381) centre (64.23, 29.365) ccw
  arc A383 (64.8919, 29.9731) -> (64.8381, 30.0269) centre (64.865, 30) ccw
  line L131 (62.325, 27.46) -> (61.69, 28.095)
  arc A384 (61.7169, 28.1219) -> (61.6631, 28.0681) centre (61.69, 28.095) ccw
  arc A385 (62.2981, 27.4331) -> (62.3519, 27.4869) centre (62.325, 27.46) ccw
  line L132 (61.69, 29.365) -> (62.325, 30)
  arc A386 (62.3519, 29.9731) -> (62.2981, 30.0269) centre (62.325, 30) ccw
  arc A387 (61.6631, 29.3919) -> (61.7169, 29.3381) centre (61.69, 29.365) ccw
  line L133 (63.595, 30) -> (62.325, 30)
  arc A388 (62.325, 30.0381) -> (62.325, 29.9619) centre (62.325, 30) ccw
  arc A389 (63.595, 29.9619) -> (63.595, 30.0381) centre (63.595, 30) ccw
  line L134 (66.77, 28.095) -> (67.405, 27.46)
  arc A390 (67.3781, 27.4331) -> (67.4319, 27.4869) centre (67.405, 27.46) ccw
  arc A391 (66.7969, 28.1219) -> (66.7431, 28.0681) centre (66.77, 28.095) ccw
  line L135 (67.405, 27.46) -> (68.675, 27.46)
  arc A392 (68.675, 27.4219) -> (68.675, 27.4981) centre (68.675, 27.46) ccw
  arc A393 (67.405, 27.4981) -> (67.405, 27.4219) centre (67.405, 27.46) ccw
  line L136 (68.675, 27.46) -> (69.31, 28.095)
  arc A394 (69.3369, 28.0681) -> (69.2831, 28.1219) centre (69.31, 28.095) ccw
  arc A395 (68.6481, 27.4869) -> (68.7019, 27.4331) centre (68.675, 27.46) ccw
  line L137 (69.31, 29.365) -> (68.675, 30)
  arc A396 (68.7019, 30.0269) -> (68.6481, 29.9731) centre (68.675, 30) ccw
  arc A397 (69.2831, 29.3381) -> (69.3369, 29.3919) centre (69.31, 29.365) ccw
  line L138 (68.675, 30) -> (67.405, 30)
  arc A398 (67.405, 30.0381) -> (67.405, 29.9619) centre (67.405, 30) ccw
  arc A399 (68.675, 29.9619) -> (68.675, 30.0381) centre (68.675, 30) ccw
  line L139 (67.405, 30) -> (66.77, 29.365)
  arc A400 (66.7431, 29.3919) -> (66.7969, 29.3381) centre (66.77, 29.365) ccw
  arc A401 (67.4319, 29.9731) -> (67.3781, 30.0269) centre (67.405, 30) ccw
  line L140 (69.945, 27.46) -> (71.215, 27.46)
  arc A402 (71.215, 27.4219) -> (71.215, 27.4981) centre (71.215, 27.46) ccw
  arc A403 (69.945, 27.4981) -> (69.945, 27.4219) centre (69.945, 27.46) ccw
  line L141 (71.215, 27.46) -> (71.85, 28.095)
  arc A404 (71.8769, 28.0681) -> (71.8231, 28.1219) centre (71.85, 28.095) ccw
  arc A405 (71.1881, 27.4869) -> (71.2419, 27.4331) centre (71.215, 27.46) ccw
  line L142 (71.85, 29.365) -> (71.215, 30)
  arc A406 (71.2419, 30.0269) -> (71.1881, 29.9731) centre (71.215, 30) ccw
  arc A407 (71.8231, 29.3381) -> (71.8769, 29.3919) centre (71.85, 29.365) ccw
  line L143 (71.85, 28.095) -> (72.485, 27.46)
  arc A408 (72.4581, 27.4331) -> (72.5119, 27.4869) centre (72.485, 27.46) ccw
  arc A409 (71.8769, 28.1219) -> (71.8231, 28.0681) centre (71.85, 28.095) ccw
  line L144 (72.485, 27.46) -> (73.755, 27.46)
  arc A410 (73.755, 27.4219) -> (73.755, 27.4981) centre (73.755, 27.46) ccw
  arc A411 (72.485, 27.4981) -> (72.485, 27.4219) centre (72.485, 27.46) ccw
  line L145 (73.755, 27.46) -> (74.39, 28.095)
  arc A412 (74.4169, 28.0681) -> (74.3631, 28.1219) centre (74.39, 28.095) ccw
  arc A413 (73.7281, 27.4869) -> (73.7819, 27.4331) centre (73.755, 27.46) ccw
  line L146 (74.39, 29.365) -> (73.755, 30)
  arc A414 (73.7819, 30.0269) -> (73.7281, 29.9731) centre (73.755, 30) ccw
  arc A415 (74.3631, 29.3381) -> (74.4169, 29.3919) centre (74.39, 29.365) ccw
  line L147 (73.755, 30) -> (72.485, 30)
  arc A416 (72.485, 30.0381) -> (72.485, 29.9619) centre (72.485, 30) ccw
  arc A417 (73.755, 29.9619) -> (73.755, 30.0381) centre (73.755, 30) ccw
  line L148 (72.485, 30) -> (71.85, 29.365)
  arc A418 (71.8231, 29.3919) -> (71.8769, 29.3381) centre (71.85, 29.365) ccw
  arc A419 (72.5119, 29.9731) -> (72.4581, 30.0269) centre (72.485, 30) ccw
  line L149 (69.945, 27.46) -> (69.31, 28.095)
  arc A420 (69.3369, 28.1219) -> (69.2831, 28.0681) centre (69.31, 28.095) ccw
  arc A421 (69.9181, 27.4331) -> (69.9719, 27.4869) centre (69.945, 27.46) ccw
  line L150 (69.31, 29.365) -> (69.945, 30)
  arc A422 (69.9719, 29.9731) -> (69.9181, 30.0269) centre (69.945, 30) ccw
  arc A423 (69.2831, 29.3919) -> (69.3369, 29.3381) centre (69.31, 29.365) ccw
  line L151 (71.215, 30) -> (69.945, 30)
  arc A424 (69.945, 30.0381) -> (69.945, 29.9619) centre (69.945, 30) ccw
  arc A425 (71.215, 29.9619) -> (71.215, 30.0381) centre (71.215, 30) ccw
  line L152 (74.39, 28.095) -> (75.025, 27.46)
  arc A426 (74.9981, 27.4331) -> (75.0519, 27.4869) centre (75.025, 27.46) ccw
  arc A427 (74.4169, 28.1219) -> (74.3631, 28.0681) centre (74.39, 28.095) ccw
  line L153 (75.025, 27.46) -> (76.295, 27.46)
  arc A428 (76.295, 27.4219) -> (76.295, 27.4981) centre (76.295, 27.46) ccw
  arc A429 (75.025, 27.4981) -> (75.025, 27.4219) centre (75.025, 27.46) ccw
  line L154 (76.295, 27.46) -> (76.93, 28.095)
  arc A430 (76.9569, 28.0681) -> (76.9031, 28.1219) centre (76.93, 28.095) ccw
  arc A431 (76.2681, 27.4869) -> (76.3219, 27.4331) centre (76.295, 27.46) ccw
  line L155 (76.93, 29.365) -> (76.295, 30)
  arc A432 (76.3219, 30.0269) -> (76.2681, 29.9731) centre (76.295, 30) ccw
  arc A433 (76.9031, 29.3381) -> (76.9569, 29.3919) centre (76.93, 29.365) ccw
  line L156 (76.295, 30) -> (75.025, 30)
  arc A434 (75.025, 30.0381) -> (75.025, 29.9619) centre (75.025, 30) ccw
  arc A435 (76.295, 29.9619) -> (76.295, 30.0381) centre (76.295, 30) ccw
  line L157 (75.025, 30) -> (74.39, 29.365)
  arc A436 (74.3631, 29.3919) -> (74.4169, 29.3381) centre (74.39, 29.365) ccw
  arc A437 (75.0519, 29.9731) -> (74.9981, 30.0269) centre (75.025, 30) ccw
  line L158 (76.93, 28.095) -> (77.565, 27.46)
  arc A438 (77.5381, 27.4331) -> (77.5919, 27.4869) centre (77.565, 27.46) ccw
  arc A439 (76.9569, 28.1219) -> (76.9031, 28.0681) centre (76.93, 28.095) ccw
  line L159 (77.565, 27.46) -> (78.835, 27.46)
  arc A440 (78.835, 27.4219) -> (78.835, 27.4981) centre (78.835, 27.46) ccw
  arc A441 (77.565, 27.4981) -> (77.565, 27.4219) centre (77.565, 27.46) ccw
  line L160 (79.47, 28.095) -> (79.47, 29.365)
  arc A442 (79.5081, 29.365) -> (79.4319, 29.365) centre (79.47, 29.365) ccw
  arc A443 (79.4319, 28.095) -> (79.5081, 28.095) centre (79.47, 28.095) ccw
  line L161 (78.835, 27.46) -> (79.47, 28.095)
  arc A444 (79.4969, 28.0681) -> (79.4431, 28.1219) centre (79.47, 28.095) ccw
  arc A445 (78.8081, 27.4869) -> (78.8619, 27.4331) centre (78.835, 27.46) ccw
  line L162 (79.47, 29.365) -> (78.835, 30)
  arc A446 (78.8619, 30.0269) -> (78.8081, 29.9731) centre (78.835, 30) ccw
  arc A447 (79.4431, 29.3381) -> (79.4969, 29.3919) centre (79.47, 29.365) ccw
  line L163 (78.835, 30) -> (77.565, 30)
  arc A448 (77.565, 30.0381) -> (77.565, 29.9619) centre (77.565, 30) ccw
  arc A449 (78.835, 29.9619) -> (78.835, 30.0381) centre (78.835, 30) ccw
  line L164 (77.565, 30) -> (76.93, 29.365)
  arc A450 (76.9031, 29.3919) -> (76.9569, 29.3381) centre (76.93, 29.365) ccw
  arc A451 (77.5919, 29.9731) -> (77.5381, 30.0269) centre (77.565, 30) ccw
  line L165 (47.9105, 31.3335) -> (47.593, 31.5875)
  arc A452 (47.6128, 31.6123) -> (47.5732, 31.5627) centre (47.593, 31.5875) ccw
  arc A453 (47.8907, 31.3087) -> (47.9303, 31.3583) centre (47.9105, 31.3335) ccw
  line L166 (47.593, 31.5875) -> (47.593, 30.4445)
  arc A454 (47.5613, 30.4445) -> (47.6248, 30.4445) centre (47.5931, 30.4445) ccw
  arc A455 (47.6248, 31.5875) -> (47.5613, 31.5875) centre (47.5931, 31.5875) ccw
  line L167 (47.9105, 30.4445) -> (47.2755, 30.4445)
  arc A456 (47.2755, 30.4763) -> (47.2755, 30.4128) centre (47.2755, 30.4445) ccw
  arc A457 (47.9105, 30.4128) -> (47.9105, 30.4763) centre (47.9105, 30.4445) ccw
  line L168 (78.8985, 26.7615) -> (78.581, 27.0155)
  arc A458 (78.6008, 27.0403) -> (78.5612, 26.9907) centre (78.581, 27.0155) ccw
  arc A459 (78.8787, 26.7367) -> (78.9183, 26.7863) centre (78.8985, 26.7615) ccw
  line L169 (78.581, 27.0155) -> (78.581, 25.8725)
  arc A460 (78.5493, 25.8725) -> (78.6128, 25.8725) centre (78.5811, 25.8725) ccw
  arc A461 (78.6128, 27.0155) -> (78.5493, 27.0155) centre (78.5811, 27.0155) ccw
  line L170 (78.8985, 25.8725) -> (78.2635, 25.8725)
  arc A462 (78.2635, 25.9043) -> (78.2635, 25.8408) centre (78.2635, 25.8726) ccw
  arc A463 (78.8985, 25.8408) -> (78.8985, 25.9043) centre (78.8985, 25.8726) ccw
  line L171 (77.7555, 25.8725) -> (77.438, 25.8725)
  arc A464 (77.438, 25.9043) -> (77.438, 25.8408) centre (77.438, 25.8726) ccw
  arc A465 (77.7555, 25.8408) -> (77.7555, 25.9043) centre (77.7555, 25.8726) ccw
  arc A466 (77.438, 26.5075) -> (77.438, 25.8725) centre (77.438, 26.19) ccw
  arc A467 (77.438, 26.4758) -> (77.438, 26.5392) centre (77.438, 26.5075) ccw
  arc A468 (77.438, 25.8408) -> (77.438, 25.9043) centre (77.438, 25.8726) ccw
  line L172 (77.7555, 27.0155) -> (77.3745, 27.0155)
  arc A469 (77.3745, 27.0473) -> (77.3745, 26.9838) centre (77.3745, 27.0155) ccw
  arc A470 (77.7555, 26.9838) -> (77.7555, 27.0473) centre (77.7555, 27.0155) ccw
  arc A471 (77.3745, 27.0155) -> (77.3745, 26.5075) centre (77.3745, 26.7615) ccw
  arc A472 (77.3745, 26.9838) -> (77.3745, 27.0473) centre (77.3745, 27.0155) ccw
  arc A473 (77.3745, 26.4758) -> (77.3745, 26.5392) centre (77.3745, 26.5075) ccw
  line L173 (77.3745, 26.5075) -> (77.6285, 26.5075)
  arc A474 (77.6285, 26.4758) -> (77.6285, 26.5392) centre (77.6285, 26.5075) ccw
  arc A475 (77.3745, 26.5392) -> (77.3745, 26.4758) centre (77.3745, 26.5075) ccw
  line L174 (92.13, 32.69) -> (92.13, 27.61)
  arc A476 (92.0983, 27.61) -> (92.1618, 27.61) centre (92.1301, 27.61) ccw
  arc A477 (92.1618, 32.69) -> (92.0983, 32.69) centre (92.1301, 32.69) ccw
  line L175 (92.13, 27.61) -> (90.86, 27.61)
  arc A478 (90.86, 27.6418) -> (90.86, 27.5783) centre (90.86, 27.6101) ccw
  arc A479 (92.13, 27.5783) -> (92.13, 27.6418) centre (92.13, 27.6101) ccw
  line L176 (90.86, 27.61) -> (83.24, 27.61)
  arc A480 (83.24, 27.6418) -> (83.24, 27.5783) centre (83.24, 27.6101) ccw
  arc A481 (90.86, 27.5783) -> (90.86, 27.6418) centre (90.86, 27.6101) ccw
  line L177 (83.24, 27.61) -> (81.97, 27.61)
  arc A482 (81.97, 27.6418) -> (81.97, 27.5783) centre (81.97, 27.6101) ccw
  arc A483 (83.24, 27.5783) -> (83.24, 27.6418) centre (83.24, 27.6101) ccw
  line L178 (81.97, 27.61) -> (81.97, 32.69)
  arc A484 (82.0018, 32.69) -> (81.9382, 32.69) centre (81.97, 32.69) ccw
  arc A485 (81.9382, 27.61) -> (82.0018, 27.61) centre (81.97, 27.61) ccw
  line L179 (81.97, 32.69) -> (92.13, 32.69)
  arc A486 (92.13, 32.6583) -> (92.13, 32.7218) centre (92.13, 32.69) ccw
  arc A487 (81.97, 32.7218) -> (81.97, 32.6583) centre (81.97, 32.69) ccw
  line L180 (90.86, 27.61) -> (90.86, 28.88)
  arc A488 (90.8918, 28.88) -> (90.8282, 28.88) centre (90.86, 28.88) ccw
  arc A489 (90.8282, 27.61) -> (90.8918, 27.61) centre (90.86, 27.61) ccw
  line L181 (90.86, 28.88) -> (83.24, 28.88)
  arc A490 (83.24, 28.9118) -> (83.24, 28.8483) centre (83.24, 28.88) ccw
  arc A491 (90.86, 28.8483) -> (90.86, 28.9118) centre (90.86, 28.88) ccw
  line L182 (83.24, 28.88) -> (83.24, 27.61)
  arc A492 (83.2083, 27.61) -> (83.2718, 27.61) centre (83.24, 27.61) ccw
  arc A493 (83.2718, 28.88) -> (83.2083, 28.88) centre (83.24, 28.88) ccw
  line L183 (35.695, 31.885) -> (36.695, 31.885)
  line L184 (36.695, 31.885) -> (36.695, 32.885)
  line L185 (36.695, 32.885) -> (35.695, 32.885)
  line L186 (35.695, 32.885) -> (35.695, 31.885)
  line L187 (33.6804, 33.3756) -> (33.6804, 31.3944)
  arc A494 (33.1851, 31.3944) -> (34.1757, 31.3944) centre (33.6804, 31.3944) ccw
  arc A495 (34.1757, 33.3756) -> (33.1851, 33.3756) centre (33.6804, 33.3756) ccw
  line L188 (33.6804, 33.3756) -> (33.6804, 31.3944)
  arc A496 (33.1851, 31.3944) -> (34.1757, 31.3944) centre (33.6804, 31.3944) ccw
  arc A497 (34.1757, 33.3756) -> (33.1851, 33.3756) centre (33.6804, 33.3756) ccw
  line L189 (38.7096, 33.3756) -> (38.7096, 31.3944)
  arc A498 (38.2143, 31.3944) -> (39.2049, 31.3944) centre (38.7096, 31.3944) ccw
  arc A499 (39.2049, 33.3756) -> (38.2143, 33.3756) centre (38.7096, 33.3756) ccw
  line L190 (38.7096, 33.3756) -> (38.7096, 31.3944)
  arc A500 (38.2143, 31.3944) -> (39.2049, 31.3944) centre (38.7096, 31.3944) ccw
  arc A501 (39.2049, 33.3756) -> (38.2143, 33.3756) centre (38.7096, 33.3756) ccw
  line L191 (50.006, 28.476) -> (50.514, 28.476)
  line L192 (50.514, 28.476) -> (50.514, 28.984)
  line L193 (50.514, 28.984) -> (50.006, 28.984)
  line L194 (50.006, 28.984) -> (50.006, 28.476)
  line L195 (47.466, 28.476) -> (47.974, 28.476)
  line L196 (47.974, 28.476) -> (47.974, 28.984)
  line L197 (47.974, 28.984) -> (47.466, 28.984)
  line L198 (47.466, 28.984) -> (47.466, 28.476)
  line L199 (52.546, 28.476) -> (53.054, 28.476)
  line L200 (53.054, 28.476) -> (53.054, 28.984)
  line L201 (53.054, 28.984) -> (52.546, 28.984)
  line L202 (52.546, 28.984) -> (52.546, 28.476)
  line L203 (57.626, 28.476) -> (58.134, 28.476)
  line L204 (58.134, 28.476) -> (58.134, 28.984)
  line L205 (58.134, 28.984) -> (57.626, 28.984)
  line L206 (57.626, 28.984) -> (57.626, 28.476)
  line L207 (55.086, 28.476) -> (55.594, 28.476)
  line L208 (55.594, 28.476) -> (55.594, 28.984)
  line L209 (55.594, 28.984) -> (55.086, 28.984)
  line L210 (55.086, 28.984) -> (55.086, 28.476)
  line L211 (60.166, 28.476) -> (60.674, 28.476)
  line L212 (60.674, 28.476) -> (60.674, 28.984)
  line L213 (60.674, 28.984) -> (60.166, 28.984)
  line L214 (60.166, 28.984) -> (60.166, 28.476)
  line L215 (65.246, 28.476) -> (65.754, 28.476)
  line L216 (65.754, 28.476) -> (65.754, 28.984)
  line L217 (65.754, 28.984) -> (65.246, 28.984)
  line L218 (65.246, 28.984) -> (65.246, 28.476)
  line L219 (62.706, 28.476) -> (63.214, 28.476)
  line L220 (63.214, 28.476) -> (63.214, 28.984)
  line L221 (63.214, 28.984) -> (62.706, 28.984)
  line L222 (62.706, 28.984) -> (62.706, 28.476)
  line L223 (67.786, 28.476) -> (68.294, 28.476)
  line L224 (68.294, 28.476) -> (68.294, 28.984)
  line L225 (68.294, 28.984) -> (67.786, 28.984)
  line L226 (67.786, 28.984) -> (67.786, 28.476)
  line L227 (72.866, 28.476) -> (73.374, 28.476)
  line L228 (73.374, 28.476) -> (73.374, 28.984)
  line L229 (73.374, 28.984) -> (72.866, 28.984)
  line L230 (72.866, 28.984) -> (72.866, 28.476)
  line L231 (70.326, 28.476) -> (70.834, 28.476)
  line L232 (70.834, 28.476) -> (70.834, 28.984)
  line L233 (70.834, 28.984) -> (70.326, 28.984)
  line L234 (70.326, 28.984) -> (70.326, 28.476)
  line L235 (75.406, 28.476) -> (75.914, 28.476)
  line L236 (75.914, 28.476) -> (75.914, 28.984)
  line L237 (75.914, 28.984) -> (75.406, 28.984)
  line L238 (75.406, 28.984) -> (75.406, 28.476)
  line L239 (77.946, 28.476) -> (78.454, 28.476)
  line L240 (78.454, 28.476) -> (78.454, 28.984)
  line L241 (78.454, 28.984) -> (77.946, 28.984)
  line L242 (77.946, 28.984) -> (77.946, 28.476)